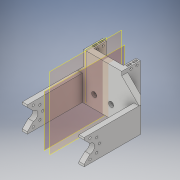
# Autodesk Inventor part: lower_head
Saved by Autodesk Inventor 2018 (Build 220112000, 112)
## iProperties
Created: 2019-07-26
Part Number: lower_head
Material: Generic
Document SubType Name: Modeling
Designer: Jasper
Density: 1 g/cm^3
Appearance: Default
Author: Jasper
Autodesk Inventor part; units mm, degrees
ref_plane "YZ Plane" through (0, 0, 0) normal (1, 0, 0) x (0, 1, 0)
ref_plane "XZ Plane" through (0, 0, 0) normal (0, 1, 0) x (-1, 0, 0)
ref_plane "XY Plane" through (0, 0, 0) normal (0, 0, 1) x (1, 0, 0)
ref_plane "Work Plane1" through (0, 0, 0) normal (0, 0, 1) x (1, 0, 0)
sketch "Sketch1" plane through (0, 0, 0) normal (0, 0, 1) x (1, 0, 0)
  spline S0 degree 3 poles (24.945, 36.948) (24.9657, 36.9478) (24.9864, 36.9481) (25.0138, 36.949) (25.0204, 36.9492) (25.0506, 36.9504) (25.0741, 36.9518) (25.1459, 36.9572) (25.1935, 36.9625) (25.3334, 36.9824) (25.4011, 36.9974) (25.4283, 36.9999) (25.4303, 37) (25.4323, 37) knots 0 0 0 0 0.104821 0.104821 0.138462 0.138462 0.257669 0.257669 0.503006 0.503006 0.968716 0.968716 1 1 1 1 construction
  spline S1 degree 3 poles (24.4578, 37) (24.4582, 37) (24.4584, 37) (24.4781, 36.9997) (24.546, 36.9843) (24.6885, 36.9635) (24.7373, 36.9579) (24.8123, 36.952) (24.8376, 36.9505) (24.8705, 36.9492) (24.878, 36.9489) (24.9054, 36.9481) (24.9252, 36.9478) (24.945, 36.948) knots 0 0 0 0 0.004459 0.004459 0.478269 0.478269 0.731877 0.731877 0.860778 0.860778 0.899168 0.899168 1 1 1 1 construction
  line L0 (24.4578, 37) -> (12.2323, 37) construction
  spline S2 degree 3 poles (11.745, 36.948) (11.7637, 36.9478) (11.7823, 36.9481) (11.8086, 36.9488) (11.8162, 36.949) (11.8484, 36.9503) (11.873, 36.9517) (11.9459, 36.9572) (11.9935, 36.9625) (12.1334, 36.9824) (12.2011, 36.9975) (12.2283, 36.9999) (12.2303, 37) (12.2323, 37) knots 0 0 0 0 0.094473 0.094473 0.133014 0.133014 0.257683 0.257683 0.503048 0.503048 0.968909 0.968909 1 1 1 1 construction
  spline S3 degree 3 poles (11.2578, 37) (11.2582, 37) (11.2584, 37) (11.278, 36.9997) (11.346, 36.9843) (11.4885, 36.9635) (11.5373, 36.9579) (11.611, 36.9521) (11.635, 36.9507) (11.6654, 36.9494) (11.6718, 36.9491) (11.7005, 36.9482) (11.7227, 36.9478) (11.745, 36.948) knots 0 0 0 0 0.004371 0.004371 0.478215 0.478215 0.731915 0.731915 0.854103 0.854103 0.886738 0.886738 1 1 1 1 construction
  line L1 (11.2578, 37) -> (9.1048, 37) construction
  line L2 (9.1048, 37) -> (0.945, 37) construction
  line L3 (0.945, 2.1131) -> (0.945, 37) construction
  line L4 (0.9925, 0.3) -> (0.945, 2.1131) construction
  line L5 (27.8975, 0.3) -> (0.9925, 0.3) construction
  line L6 (27.945, 2.1131) -> (27.8975, 0.3) construction
  line L7 (27.945, 37) -> (27.945, 2.1131) construction
  line L8 (27.945, 37) -> (27.5852, 37) construction
  line L9 (27.5852, 37) -> (25.4323, 37) construction
  circle A0 centre (4.445, 3) radius 1.7561 construction
  circle A1 centre (8.445, 4.5) radius 1.1544 construction
  circle A2 centre (20.445, 4.5) radius 1.1544 construction
  circle A3 centre (24.445, 3) radius 1.7561 construction
  line L10 (20.445, 29.1974) -> (16.2772, 29.1974) construction
  arc A4 (20.445, 23.8026) -> (20.445, 29.1974) centre (20.445, 26.5) ccw construction
  line L11 (15.54, 23.8026) -> (20.445, 23.8026) construction
  arc A5 (13.35, 23.8026) -> (15.54, 23.8026) centre (14.445, 26.7) ccw construction
  line L12 (8.445, 23.8026) -> (13.35, 23.8026) construction
  arc A6 (8.445, 29.1974) -> (8.445, 23.8026) centre (8.445, 26.5) ccw construction
  line L13 (12.6128, 29.1974) -> (8.445, 29.1974) construction
  arc A7 (16.2772, 29.1974) -> (12.6128, 29.1974) centre (14.445, 26.7) ccw construction
  line L14 (1.0679, 41.7079) -> (27.8221, 41.7079) construction
  line L15 (36.945, -12) -> (-8.055, -12)
  line L16 (-8.055, -12) -> (-8.055, 65.4)
  line L17 (-8.055, 65.4) -> (36.945, 65.4)
  line L18 (36.945, 65.4) -> (36.945, -12)
  line L19 (36.945, -12) -> (-8.055, 65.4) construction
  line L20 (-8.055, -12) -> (36.945, 65.4) construction
  point P0 (0, 0)
  point P1 (14.445, -12)
  dimension "d0" = 45
  dimension "d13" = 77.4
  constraints: 12 end point, 3 midpoint, 2 parallel, 1 horizontal, 1 perpendicular
  measures "d0" distance of L16.end L17.end
  measures "d13" distance between parallel lines of L15 L17
extrude "Extrusion1" add sketch "Sketch1" along normal blind 5
sketch "Sketch4" plane through (0, 0, 5) normal (0, 0, 1) x (1, 0, 0)
  line L0 (-8.055, -12) -> (36.945, -12) construction
  line L1 (36.945, -12) -> (36.945, 65.4) construction
  line L2 (36.945, 65.4) -> (-8.055, 65.4) construction
  line L3 (-8.055, 65.4) -> (-8.055, -12) construction
  line L4 (36.945, -12) -> (14.445, -12) construction
  line L5 (14.445, -12) -> (14.445, 23) construction
  line L6 (-15.555, -12) -> (44.445, -12)
  line L7 (44.445, -12) -> (44.445, 58)
  line L8 (44.445, 58) -> (-15.555, 58)
  line L9 (-15.555, 58) -> (-15.555, -12)
  line L10 (-15.555, -12) -> (44.445, 58) construction
  line L11 (44.445, -12) -> (-15.555, 58) construction
  line L12 (44.445, 58) -> (57.445, 58)
  line L13 (57.445, 58) -> (57.445, -12)
  line L14 (57.445, -12) -> (44.445, -12)
  line L15 (44.445, -12) -> (44.445, 58)
  point P0 (0, 0)
  dimension "d9" = 22.5
  dimension "d10" = 35
  dimension "d11" = 60
  dimension "d12" = 70
  dimension "d14" = 13
  dimension "d15" = 70
  constraints: 24 end point, 4 parallel, 3 midpoint, 3 perpendicular, 2 horizontal
  measures "d9" distance of L0.end L4.end
  measures "d10" distance of L4.end L5.end
  measures "d11" distance between parallel lines of L9 L7
  measures "d12" distance between parallel lines of L6 L8
  measures "d14" distance of L13.end L14.end
  measures "d15" distance of L12.end L13.end
extrude "Extrusion3" add sketch "Sketch4" along normal blind 2
sketch "Sketch5" plane through (0, 0, 7) normal (0, 0, 1) x (1, 0, 0)
  line L0 (-15.555, -12) -> (57.445, -12) construction
  line L1 (57.445, -12) -> (57.445, 58) construction
  line L2 (57.445, 58) -> (-15.555, 58) construction
  line L3 (-15.555, 58) -> (-15.555, -12) construction
  spline S0 degree 3 poles (24.945, 36.948) (24.9657, 36.9478) (24.9864, 36.9481) (25.0138, 36.949) (25.0204, 36.9492) (25.0506, 36.9504) (25.0741, 36.9518) (25.1459, 36.9572) (25.1935, 36.9625) (25.3334, 36.9824) (25.4011, 36.9974) (25.4283, 36.9999) (25.4303, 37) (25.4323, 37) knots 0 0 0 0 0.104821 0.104821 0.138462 0.138462 0.257669 0.257669 0.503006 0.503006 0.968716 0.968716 1 1 1 1 construction
  spline S1 degree 3 poles (24.4578, 37) (24.4582, 37) (24.4584, 37) (24.4781, 36.9997) (24.546, 36.9843) (24.6885, 36.9635) (24.7373, 36.9579) (24.8123, 36.952) (24.8376, 36.9505) (24.8705, 36.9492) (24.878, 36.9489) (24.9054, 36.9481) (24.9252, 36.9478) (24.945, 36.948) knots 0 0 0 0 0.004459 0.004459 0.478269 0.478269 0.731877 0.731877 0.860778 0.860778 0.899168 0.899168 1 1 1 1 construction
  line L4 (24.4578, 37) -> (12.2323, 37) construction
  spline S2 degree 3 poles (11.745, 36.948) (11.7637, 36.9478) (11.7823, 36.9481) (11.8086, 36.9488) (11.8162, 36.949) (11.8484, 36.9503) (11.873, 36.9517) (11.9459, 36.9572) (11.9935, 36.9625) (12.1334, 36.9824) (12.2011, 36.9975) (12.2283, 36.9999) (12.2303, 37) (12.2323, 37) knots 0 0 0 0 0.094473 0.094473 0.133014 0.133014 0.257683 0.257683 0.503048 0.503048 0.968909 0.968909 1 1 1 1 construction
  spline S3 degree 3 poles (11.2578, 37) (11.2582, 37) (11.2584, 37) (11.278, 36.9997) (11.346, 36.9843) (11.4885, 36.9635) (11.5373, 36.9579) (11.611, 36.9521) (11.635, 36.9507) (11.6654, 36.9494) (11.6718, 36.9491) (11.7005, 36.9482) (11.7227, 36.9478) (11.745, 36.948) knots 0 0 0 0 0.004371 0.004371 0.478215 0.478215 0.731915 0.731915 0.854103 0.854103 0.886738 0.886738 1 1 1 1 construction
  line L5 (11.2578, 37) -> (9.1048, 37) construction
  line L6 (9.1048, 37) -> (0.945, 37) construction
  line L7 (0.945, 2.1131) -> (0.945, 37) construction
  line L8 (0.9925, 0.3) -> (0.945, 2.1131) construction
  line L9 (27.8975, 0.3) -> (0.9925, 0.3) construction
  line L10 (27.945, 2.1131) -> (27.8975, 0.3) construction
  line L11 (27.945, 37) -> (27.945, 2.1131) construction
  line L12 (27.945, 37) -> (27.5852, 37) construction
  line L13 (27.5852, 37) -> (25.4323, 37) construction
  circle A0 centre (4.445, 3) radius 1.7561 construction
  circle A1 centre (8.445, 4.5) radius 1.1544 construction
  circle A2 centre (20.445, 4.5) radius 1.1544 construction
  circle A3 centre (24.445, 3) radius 1.7561 construction
  line L14 (20.445, 29.1974) -> (16.2772, 29.1974) construction
  arc A4 (20.445, 23.8026) -> (20.445, 29.1974) centre (20.445, 26.5) ccw construction
  line L15 (15.54, 23.8026) -> (20.445, 23.8026) construction
  arc A5 (13.35, 23.8026) -> (15.54, 23.8026) centre (14.445, 26.7) ccw construction
  line L16 (8.445, 23.8026) -> (13.35, 23.8026) construction
  arc A6 (8.445, 29.1974) -> (8.445, 23.8026) centre (8.445, 26.5) ccw construction
  line L17 (12.6128, 29.1974) -> (8.445, 29.1974) construction
  arc A7 (16.2772, 29.1974) -> (12.6128, 29.1974) centre (14.445, 26.7) ccw construction
  line L18 (4.445, 3) -> (-15.555, 3) construction
  line L19 (-15.555, 58) -> (-15.555, -12)
  line L20 (-15.555, 3) -> (-0.555, 3) construction
  line L21 (-15.555, -12) -> (-9.555, -12)
  line L22 (-9.555, -12) -> (-9.555, 18)
  line L23 (-9.555, 18) -> (-15.555, 18)
  line L24 (-15.555, 18) -> (-15.555, -12)
  line L25 (57.445, -12) -> (20.945, -12) construction
  line L26 (36.945, -12) -> (-8.055, -12)
  line L27 (20.945, -12) -> (20.945, 58) construction
  line L28 (57.445, -12) -> (51.445, -12)
  line L29 (51.445, -12) -> (51.445, 18)
  line L30 (51.445, 18) -> (57.445, 18)
  line L31 (57.445, 18) -> (57.445, -12)
  point P0 (0, 0)
  point P1 (18.0626, 18.5071)
  dimension "d24" = 6
  dimension "d25" = 30
  dimension "d26" = 36.5
  dimension "d27" = 70
  dimension "d28" = 90
  constraints: 24 end point, 3 horizontal, 3 symmetric about line, 2 parallel, 2 perpendicular, 2 point on line, 1 other
  measures "d24" distance of L23.end L22.end
  measures "d25" distance of L22.end L21.end
  measures "d26" distance of L0.end L25.end
  measures "d27" distance of L25.end L27.end
  measures "d28" angle of L25 L27
sketch "Sketch6" plane through (0, 0, 0) normal (0, 0, -1) x (-1, 0, 0)
  line L0 (-36.945, -12) -> (8.055, -12) construction
  line L1 (8.055, -12) -> (8.055, 65.4) construction
  line L2 (8.055, 65.4) -> (-36.945, 65.4) construction
  line L3 (-36.945, 65.4) -> (-36.945, -12) construction
  line L4 (-36.945, -12) -> (8.055, -12)
  line L5 (8.055, -12) -> (8.055, -7)
  line L6 (8.055, -7) -> (-36.945, -7)
  line L7 (-36.945, -7) -> (-36.945, -12)
  point P0 (0, 0)
  dimension "d20" = 45
  dimension "d21" = 5
  constraints: 8 end point, 2 parallel, 1 horizontal, 1 perpendicular
  measures "d20" distance of L6.end L5.end
  measures "d21" distance of L5.end L4.end
extrude "Extrusion4" cut sketch "Sketch6" against normal blind 5
extrude "Extrusion5" add sketch "Sketch5" along normal blind 65
sketch "Sketch8" plane through (0, 0, 5) normal (0, 0, -1) x (-1, 0, 0)
  line L0 (-36.945, -7) -> (-36.945, 58) projected
  line L1 (-57.445, 58) -> (-36.945, 58) projected
  line L2 (-57.445, -12) -> (-57.445, 58) projected
  line L3 (-57.445, 18) -> (-57.445, 58) projected
  line L4 (-57.445, 58) -> (-36.945, 58)
  line L5 (-36.945, 58) -> (-36.945, 38.5)
  line L6 (-36.945, 38.5) -> (-57.445, 38.5)
  line L7 (-57.445, 38.5) -> (-57.445, 58)
  line L8 (8.055, 58) -> (8.055, -7) projected
  line L9 (-36.945, -7) -> (8.055, -7) projected
  line L10 (15.555, -12) -> (-57.445, -12) projected
  line L11 (15.555, 58) -> (15.555, -12) projected
  line L12 (8.055, 58) -> (15.555, 58) projected
  point P0 (0, 0)
  dimension "d31" = 20.5
  dimension "d32" = 19.5
  constraints: 8 end point, 2 parallel, 1 horizontal, 1 perpendicular
  measures "d31" distance of L5.end L6.end
  measures "d32" distance of L4.end L5.end
extrude "Extrusion6" cut sketch "Sketch8" against normal up to surface (2 mm away) contours L6 L2 L1 L0
chamfer "Chamfer1" distance 20.5 angle 45 1 edges at (57.445, 38.5, 6)
sketch "Sketch9" plane through (57.445, -12, 72) normal (1, 0, 0) x (0, 0, -1)
  line L0 (0, 30) -> (0, 15) construction
  line L1 (0, 30) -> (0, 0) construction
  line L2 (0, 15) -> (7, 15) construction
  circle A0 centre (7, 15) radius 5.5
  line L3 (7, 15) -> (7, 26) construction
  line L4 (7, 15) -> (18, 15) construction
  circle A1 centre (7, 26) radius 1.35
  circle A2 centre (14.7782, 22.7782) radius 1.35
  circle A3 centre (18, 15) radius 1.35
  circle A4 centre (14.7782, 7.2218) radius 1.35
  circle A5 centre (7, 4) radius 1.35
  line L5 (7, 20.5) -> (0, 27.5)
  line L6 (7, 20.5) -> (16.8995, 20.5) construction
  line L7 (7, 9.5) -> (0, 2.5)
  line L8 (7, 20.5) -> (7, 9.5)
  line L9 (0, 27.5) -> (0, 2.5)
  point P0 (72, 12)
  dimension "d47" = 15
  dimension "d48" = 7
  dimension "d49" = 11
  dimension "d50" = 11
  dimension "d51" = 90
  dimension "d52" = 2.7
  dimension "d55" = 180
  dimension "d57" = 135
  constraints: 18 end point, 6 centre point, 2 coincident, 2 collinear, 2 equal length, 2 horizontal, 2 midpoint, 2 symmetric about line, 1 perpendicular, 1 point on line, 1 vertical, 9 other
  measures "d47" distance of L0.start L0.end
  measures "d48" distance of L0.end L2.end
  measures "d49" diameter of A0
  measures "d50" distance of L3.start L3.end
  measures "d51" angle of L4 L3
  measures "d52" diameter of A1
  measures "d57" angle of L6 L5
extrude "Extrusion7" cut sketch "Sketch9" against normal up to surface (6 mm away)
ref_plane "Work Plane2" through (20.945, -12, 7) normal (1, 0, 0) x (0, 0, -1)
mirror "Mirror1" about plane through (20.945, -12, 7) normal (1, 0, 0) of "Extrusion7"
sketch "Sketch10" plane through (0, 0, 7) normal (0, 0, 1) x (1, 0, 0)
  spline S0 degree 3 poles (24.945, 36.948) (24.9657, 36.9478) (24.9864, 36.9481) (25.0138, 36.949) (25.0204, 36.9492) (25.0506, 36.9504) (25.0741, 36.9518) (25.1459, 36.9572) (25.1935, 36.9625) (25.3334, 36.9824) (25.4011, 36.9974) (25.4283, 36.9999) (25.4303, 37) (25.4323, 37) knots 0 0 0 0 0.104821 0.104821 0.138462 0.138462 0.257669 0.257669 0.503006 0.503006 0.968716 0.968716 1 1 1 1
  spline S1 degree 3 poles (24.4578, 37) (24.4582, 37) (24.4584, 37) (24.4781, 36.9997) (24.546, 36.9843) (24.6885, 36.9635) (24.7373, 36.9579) (24.8123, 36.952) (24.8376, 36.9505) (24.8705, 36.9492) (24.878, 36.9489) (24.9054, 36.9481) (24.9252, 36.9478) (24.945, 36.948) knots 0 0 0 0 0.004459 0.004459 0.478269 0.478269 0.731877 0.731877 0.860778 0.860778 0.899168 0.899168 1 1 1 1
  line L0 (24.4578, 37) -> (12.2323, 37)
  spline S2 degree 3 poles (11.745, 36.948) (11.7637, 36.9478) (11.7823, 36.9481) (11.8086, 36.9488) (11.8162, 36.949) (11.8484, 36.9503) (11.873, 36.9517) (11.9459, 36.9572) (11.9935, 36.9625) (12.1334, 36.9824) (12.2011, 36.9975) (12.2283, 36.9999) (12.2303, 37) (12.2323, 37) knots 0 0 0 0 0.094473 0.094473 0.133014 0.133014 0.257683 0.257683 0.503048 0.503048 0.968909 0.968909 1 1 1 1
  spline S3 degree 3 poles (11.2578, 37) (11.2582, 37) (11.2584, 37) (11.278, 36.9997) (11.346, 36.9843) (11.4885, 36.9635) (11.5373, 36.9579) (11.611, 36.9521) (11.635, 36.9507) (11.6654, 36.9494) (11.6718, 36.9491) (11.7005, 36.9482) (11.7227, 36.9478) (11.745, 36.948) knots 0 0 0 0 0.004371 0.004371 0.478215 0.478215 0.731915 0.731915 0.854103 0.854103 0.886738 0.886738 1 1 1 1
  line L1 (11.2578, 37) -> (9.1048, 37)
  line L2 (9.1048, 37) -> (0.945, 37)
  line L3 (0.945, 2.1131) -> (0.945, 37)
  line L4 (0.9925, 0.3) -> (0.945, 2.1131)
  line L5 (27.8975, 0.3) -> (0.9925, 0.3)
  line L6 (27.945, 2.1131) -> (27.8975, 0.3)
  line L7 (27.945, 37) -> (27.945, 2.1131)
  line L8 (27.945, 37) -> (27.5852, 37)
  line L9 (27.5852, 37) -> (25.4323, 37)
  circle A0 centre (4.445, 3) radius 1.7561
  circle A1 centre (8.445, 4.5) radius 1.1544
  circle A2 centre (20.445, 4.5) radius 1.1544
  circle A3 centre (24.445, 3) radius 1.7561
  line L10 (20.445, 29.1974) -> (16.2772, 29.1974)
  arc A4 (20.445, 23.8026) -> (20.445, 29.1974) centre (20.445, 26.5) ccw
  line L11 (15.54, 23.8026) -> (20.445, 23.8026)
  arc A5 (13.35, 23.8026) -> (15.54, 23.8026) centre (14.445, 26.7) ccw
  line L12 (8.445, 23.8026) -> (13.35, 23.8026)
  arc A6 (8.445, 29.1974) -> (8.445, 23.8026) centre (8.445, 26.5) ccw
  line L13 (12.6128, 29.1974) -> (8.445, 29.1974)
  arc A7 (16.2772, 29.1974) -> (12.6128, 29.1974) centre (14.445, 26.7) ccw
  point P0 (0, 0)
extrude "Extrusion8" cut sketch "Sketch10" against normal up to surface (7 mm away) contours A0 | A3
sketch "Sketch11" plane through (0, 0, 7) normal (0, 0, 1) x (1, 0, 0)
  circle A0 centre (4.445, 3) radius 1.7561 construction
  circle A1 centre (24.445, 3) radius 1.7561 construction
  line L0 (-15.555, 58) -> (-15.555, 18) construction
  line L1 (-15.555, 18) -> (-9.555, 18) construction
  line L2 (-9.555, 18) -> (-9.555, -12) construction
  line L3 (-9.555, -12) -> (51.445, -12) construction
  line L4 (51.445, -12) -> (51.445, 18) construction
  line L5 (51.445, 18) -> (57.445, 18) construction
  line L6 (36.945, 38.5) -> (57.445, 18) construction
  line L7 (36.945, 38.5) -> (36.945, 58) construction
  circle A2 centre (4.445, 3) radius 3
  circle A3 centre (24.445, 3) radius 3
  line L8 (36.945, 58) -> (-15.555, 58) projected
  point P0 (0, 0)
  dimension "d62" = 6
  dimension "d63" = 6
  constraints: 2 centre point, 2 coincident
  measures "d62" diameter of A2
  measures "d63" diameter of A3
sketch "Sketch12" plane through (0, 0, 5) normal (0, 0, -1) x (-1, 0, 0)
  line L0 (8.055, 58) -> (8.055, -7) construction
  line L1 (-36.945, -7) -> (8.055, -7) construction
  line L2 (-36.945, -7) -> (-36.945, 38.5) construction
  line L3 (-57.445, 18) -> (-36.945, 38.5) construction
  line L4 (-57.445, -12) -> (-57.445, 18) construction
  line L5 (15.555, -12) -> (-57.445, -12) construction
  line L6 (15.555, 58) -> (15.555, -12) construction
  line L7 (-36.945, -7) -> (-36.945, 38.5) projected
  line L8 (-36.945, 38.5) -> (-36.945, -7)
  line L9 (-36.945, -7) -> (-57.445, -7)
  line L10 (-57.445, -7) -> (-57.445, 18)
  line L11 (-36.945, 38.5) -> (-57.445, 18) projected
  line L12 (-36.945, 38.5) -> (-57.445, 18)
  line L13 (8.055, 58) -> (15.555, 58) projected
  point P0 (0, 0)
  constraints: 8 end point, 2 collinear, 1 perpendicular, 1 point on line
extrude "Extrusion9" add sketch "Sketch12" along normal blind 5
chamfer "Chamfer5" distance 5 angle 45 1 edges at (57.445, 5.5, 0)
chamfer "Chamfer6" distance 5 angle 45 1 edges at (24.695, -7, 5)
sketch "Sketch14" plane through (0, 0, 5) normal (0, 0, -1) x (-1, 0, 0)
  line L0 (15.555, 18) -> (9.555, 18) construction
  line L1 (9.555, 18) -> (15.555, 18) construction
  line L2 (8.055, 58) -> (8.055, -12) construction
  line L3 (15.555, -12) -> (8.055, -12) construction
  line L4 (15.555, 58) -> (15.555, -12) construction
  line L5 (8.055, 58) -> (15.555, 58) construction
  line L6 (15.555, 18) -> (9.555, 18) construction
  line L7 (15.555, 18) -> (15.555, 25.5) construction
  line L8 (15.555, 58) -> (15.555, -12) construction
  line L9 (8.055, 58) -> (8.055, -12) projected
  line L10 (15.555, 25.5) -> (8.055, 25.5)
  line L11 (8.055, 25.5) -> (8.055, 58)
  line L12 (8.055, 58) -> (15.555, 58)
  line L13 (15.555, 58) -> (15.555, 25.5)
  point P0 (0, 0)
  dimension "d72" = 7.5
  constraints: 10 end point, 2 parallel, 1 horizontal, 1 perpendicular, 1 point on line
  measures "d72" distance of L6.start L7.end
extrude "Extrusion10" cut sketch "Sketch14" against normal up to surface (2 mm away)
chamfer "Chamfer7" distance 7.5 angle 45 1 edges at (-15.555, 25.5, 6)
sketch "Sketch15" plane through (0, 0, 5) normal (0, 0, -1) x (-1, 0, 0)
  line L0 (8.055, 25.5) -> (15.555, 18) projected
  line L1 (8.055, 25.5) -> (8.055, -12) projected
  line L2 (15.555, -12) -> (8.055, -12) projected
  line L3 (15.555, 18) -> (15.555, -12) projected
  point P0 (0, 0)
extrude "Extrusion11" add sketch "Sketch15" along normal blind 5
chamfer "Chamfer8" distance 5 angle 45 1 edges at (-11.805, -12, 0)
chamfer "Chamfer9" distance 5 angle 45 1 edges at (-15.555, 5.5, 0)
extrude "Extrusion12" cut sketch "Sketch11" against normal blind 3
sketch "Sketch16" plane through (0, 0, 0) normal (0, 0, -1) x (-1, 0, 0)
  line L0 (10.555, 23) -> (10.555, -7) construction
  line L1 (10.555, 23) -> (8.055, 25.5) construction
  line L2 (8.055, 25.5) -> (8.055, 65.4) construction
  line L3 (8.055, 65.4) -> (-36.945, 65.4) construction
  line L4 (-36.945, 65.4) -> (-36.945, 38.5) construction
  line L5 (-36.945, 38.5) -> (-52.445, 23) construction
  line L6 (-52.445, -7) -> (-52.445, 23) construction
  line L7 (10.555, -7) -> (-52.445, -7) construction
  circle A0 centre (-24.445, 3) radius 1.7561 construction
  circle A1 centre (-4.445, 3) radius 1.7561 construction
  line L8 (10.555, -7) -> (-52.445, -7)
  line L9 (8.055, 65.4) -> (3.055, 65.4)
  line L10 (3.055, 65.4) -> (3.055, -7)
  line L11 (3.055, -7) -> (8.055, -7)
  line L12 (8.055, -7) -> (8.055, 65.4)
  line L13 (-4.445, 3) -> (-14.445, 3) construction
  line L14 (-14.445, 3) -> (-14.445, 53) construction
  line L15 (-39.445, -7) -> (23.555, -7)
  line L16 (-36.945, 65.4) -> (-31.945, 65.4)
  line L17 (-31.945, 65.4) -> (-31.945, -7)
  line L18 (-36.945, -7) -> (-36.945, 65.4)
  line L19 (-31.945, -7) -> (-36.945, -7)
  point P0 (0, 0)
extrude "Extrusion13" add sketch "Sketch16" along normal blind 15
sketch "Sketch18" plane through (-8.055, 65.4, 5) normal (0, 1, 0) x (1, 0, 0)
  line L0 (0, 0) -> (0, 20) projected
  line L1 (45, 0) -> (0, 0) projected
  line L2 (45, 0) -> (45, 20) projected
  line L3 (40, 20) -> (45, 20) projected
  line L4 (40, 5) -> (40, 20) projected
  line L5 (5, 5) -> (40, 5) projected
  line L6 (5, 5) -> (5, 20) projected
  line L7 (0, 20) -> (5, 20) projected
  point P0 (8.055, 5)
extrude "Extrusion14" cut sketch "Sketch18" against normal blind 7.4
sketch "Sketch19" plane through (-8.055, 58, 7) normal (0, 1, 0) x (1, 0, 0)
  line L0 (0, 0) -> (0, 22) projected
  line L1 (45, 0) -> (0, 0) projected
  line L2 (45, 22) -> (45, 0) projected
  line L3 (40, 22) -> (45, 22) projected
  line L4 (40, 7) -> (40, 22) projected
  line L5 (5, 7) -> (40, 7) projected
  line L6 (5, 22) -> (5, 7) projected
  line L7 (0, 22) -> (5, 22) projected
  point P0 (8.055, 7)
extrude "Extrusion15" cut sketch "Sketch19" against normal blind 15
sketch "Sketch21" plane through (-8.055, 25.5, 0) normal (-1, 0, 0) x (0, 0, 1)
  line L0 (7, 17.5) -> (-15, 17.5) construction
  line L1 (-15, -32.5) -> (-15, 17.5) construction
  line L2 (0, -32.5) -> (-15, -32.5) construction
  line L3 (0, 0) -> (0, -32.5) construction
  line L4 (0, 0) -> (7, 0) construction
  line L5 (7, 17.5) -> (7, 0) construction
  line L6 (-15, -32.5) -> (-15, -29.5)
  line L7 (-15, -32.5) -> (-15, 17.5) projected
  line L8 (-15, -32.5) -> (-12, -32.5) construction
  line L9 (-15, -29.5) -> (-11, -29.5)
  line L10 (-11, -29.5) -> (-4, -29.5)
  line L11 (-4, -29.5) -> (-4, 14.5)
  line L12 (-4, 14.5) -> (-11, 14.5)
  circle A0 centre (-11, -29.5) radius 1.35
  circle A1 centre (-4, -29.5) radius 1.35
  circle A2 centre (-11, 14.5) radius 1.35
  circle A3 centre (-4, 14.5) radius 1.35
  point P0 (0, -25.5)
  dimension "d119" = 3
  dimension "d120" = 90
  dimension "d121" = 4
  dimension "d122" = 90
  dimension "d123" = 7
  dimension "d124" = 180
  dimension "d125" = 90
  dimension "d126" = 7
  dimension "d127" = 90
  dimension "d128" = 3
  dimension "d129" = 2.7
  dimension "d130" = 2.7
  dimension "d131" = 2.7
  dimension "d132" = 2.7
  constraints: 12 end point, 4 centre point, 4 coincident, 3 perpendicular, 2 collinear, 1 horizontal
  measures "d119" distance of L1.start L6.end
  measures "d120" angle of L8 L6
  measures "d121" distance of L6.end L9.end
  measures "d122" angle of L6 L9
  measures "d123" distance of L9.end L10.end
  measures "d124" angle of L10 L9
  measures "d125" angle of L11 L10
  measures "d126" distance of L11.end L12.end
  measures "d127" angle of L12 L11
  measures "d128" distance from line of L0 L11.end
  measures "d129" diameter of A0
  measures "d130" diameter of A1
  measures "d131" diameter of A2
  measures "d132" diameter of A3
extrude "Extrusion16" cut sketch "Sketch21" against normal up to surface (5 mm away)
ref_plane "Work Plane3" through (-4.505, 25.5, 0) normal (-1, 0, 0) x (0, 0, 1)
sketch "Sketch22" plane through (-4.505, 25.5, 0) normal (-1, 0, 0) x (0, 0, 1)
  circle A0 centre (-11, 14.5) radius 1.35 construction
  circle A1 centre (-4, 14.5) radius 1.35 construction
  circle A2 centre (-4, -29.5) radius 1.35 construction
  circle A3 centre (-11, -29.5) radius 1.35 construction
  line L0 (7, 17.5) -> (-15, 17.5) construction
  line L1 (-15, -32.5) -> (-15, 17.5) construction
  line L2 (0, -32.5) -> (-15, -32.5) construction
  line L3 (0, 0) -> (0, -32.5) construction
  line L4 (0, 0) -> (7, 0) construction
  line L5 (7, 17.5) -> (7, 0) construction
  line L6 (-11, -29.5) -> (-11, -32.5) construction
  line L7 (-11, -32.4445) -> (-13.55, -30.9722)
  line L8 (-13.55, -30.9722) -> (-13.55, -28.0278)
  line L9 (-13.55, -28.0278) -> (-11, -26.5555)
  line L10 (-11, -26.5555) -> (-8.45, -28.0278)
  line L11 (-8.45, -28.0278) -> (-8.45, -30.9722)
  line L12 (-8.45, -30.9722) -> (-11, -32.4445)
  line L13 (-13.55, -30.9722) -> (-8.45, -30.9722)
  line L14 (-8.45, -30.9722) -> (-8.45, -32.5)
  line L15 (-8.45, -32.5) -> (-13.55, -32.5)
  line L16 (-13.55, -32.5) -> (-13.55, -30.9722)
  line L17 (-15, -32.5) -> (-7.5, -32.5) construction
  line L18 (-15, -32.5) -> (-7.5, -32.5) construction
  line L19 (-7.5, -32.5) -> (-7.5, 17.5) construction
  line L20 (-15, 17.5) -> (-15, -7.5) construction
  line L21 (-15, 17.5) -> (10, 17.5) construction
  line L22 (-15, -7.5) -> (0, -7.5) construction
  line L23 (-4, -32.4445) -> (-1.45, -30.9722)
  line L24 (-1.45, -30.9722) -> (-1.45, -28.0278)
  line L25 (-1.45, -28.0278) -> (-4, -26.5555)
  line L26 (-4, -26.5555) -> (-6.55, -28.0278)
  line L27 (-6.55, -28.0278) -> (-6.55, -30.9722)
  line L28 (-6.55, -30.9722) -> (-4, -32.4445)
  line L29 (-1.45, -30.9722) -> (-6.55, -30.9722)
  line L30 (-6.55, -30.9722) -> (-6.55, -32.5)
  line L31 (-6.55, -32.5) -> (-1.45, -32.5)
  line L32 (-1.45, -32.5) -> (-1.45, -30.9722)
  circle A4 centre (-4, 14.5) radius 1.35 construction
  circle A5 centre (-11, 14.5) radius 1.35 construction
  line L33 (-11, 14.5) -> (-11, 17.5) construction
  line L34 (-11, 17.4445) -> (-13.55, 15.9722)
  line L35 (-13.55, 15.9722) -> (-13.55, 13.0278)
  line L36 (-13.55, 13.0278) -> (-11, 11.5555)
  line L37 (-11, 11.5555) -> (-8.45, 13.0278)
  line L38 (-8.45, 13.0278) -> (-8.45, 15.9722)
  line L39 (-8.45, 15.9722) -> (-11, 17.4445)
  line L40 (-13.55, 15.9722) -> (-8.45, 15.9722)
  line L41 (-8.45, 15.9722) -> (-8.45, 17.5)
  line L42 (-8.45, 17.5) -> (-13.55, 17.5)
  line L43 (-13.55, 17.5) -> (-13.55, 15.9722)
  line L44 (-15, 17.5) -> (-7.5, 17.5) construction
  line L45 (-15, 17.5) -> (-7.5, 17.5) construction
  line L46 (-1.45, 13.0278) -> (-4, 11.5555)
  line L47 (-1.45, 15.9722) -> (-1.45, 13.0278)
  line L48 (-4, 11.5555) -> (-6.55, 13.0278)
  line L49 (-6.55, 13.0278) -> (-6.55, 15.9722)
  line L50 (-1.45, 15.9722) -> (-6.55, 15.9722)
  line L51 (-6.55, 15.9722) -> (-4, 17.4445)
  line L52 (-6.55, 15.9722) -> (-6.55, 17.5)
  line L53 (-6.55, 17.5) -> (-1.45, 17.5)
  line L54 (-4, 17.4445) -> (-1.45, 15.9722)
  line L55 (-1.45, 17.5) -> (-1.45, 15.9722)
  point P0 (0, -25.5)
  dimension "d136" = 5.1
  dimension "d137" = 5.1
  dimension "d138" = 7.5
  dimension "d139" = 0
  dimension "d140" = 50
  dimension "d141" = 90
  dimension "d142" = 25
  dimension "d143" = 90
  dimension "d144" = 15
  dimension "d145" = 90
  constraints: 100 end point, 33 symmetric about line, 4 perpendicular, 4 point on line, 3 horizontal, 2 centre point, 2 coincident, 2 collinear, 2 equal length, 2 parallel, 15 other
  measures "d136" distance between parallel lines of L12 L9
  measures "d137" distance of L7.end L13.end
  measures "d138" distance of L1.start L17.end
  measures "d139" distance between parallel lines of L17 L18
  measures "d140" distance of L17.end L19.end
  measures "d141" angle of L19 L17
  measures "d142" distance of L0.end L20.end
  measures "d143" angle of L20 L21
  measures "d144" distance of L20.end L22.end
  measures "d145" angle of L22 L20
extrude "Extrusion17" cut sketch "Sketch22" along normal blind 2.1
ref_plane "Work Plane4" through (14.445, -7, -15) normal (-1, 0, 0) x (0, 0, 1)
mirror "Mirror2" about plane through (14.445, -7, -15) normal (-1, 0, 0) of "Extrusion17", "Extrusion16"
ref_plane "Work Plane5" through (14.445, -7, -15) normal (-1, 0, 0) x (0, 0, 1)
body "Solid1"
